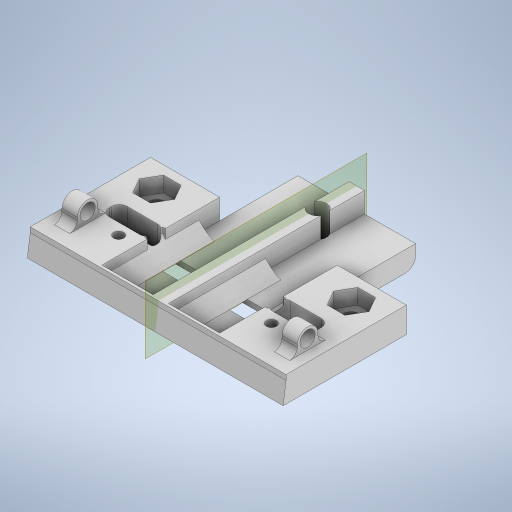
# Autodesk Inventor part: podsta
Saved by Autodesk Inventor 2023 (Build 270158000, 158)
## iProperties
Created: 2022-12-13
Part Number: podsta
Material: Generic
Document SubType Name: Modeling
Designer: komputer
Density: 1 g/cm^3
Appearance: Default
Author: komputer
Autodesk Inventor part; units mm, degrees
ref_plane "YZ Plane" through (0, 0, 0) normal (1, 0, 0) x (0, 1, 0)
ref_plane "XZ Plane" through (0, 0, 0) normal (0, 1, 0) x (-1, 0, 0)
ref_plane "XY Plane" through (0, 0, 0) normal (0, 0, 1) x (1, 0, 0)
sketch "Sketch1" plane through (0, 0, 0) normal (0, 1, 0) x (-1, 0, 0)
  line L0 (-25, -25) -> (25, -25)
  line L1 (25, -25) -> (25, 25)
  line L2 (25, 25) -> (-25, 25)
  line L3 (-25, 25) -> (-25, -25)
  point P0 (0, 0)
  dimension "d2" = 50
  dimension "d3" = 50
  constraints: 8 end point, 2 parallel, 1 horizontal, 1 perpendicular
  measures "d2" distance of L2.end L1.end
  measures "d3" distance of L1.end L0.end
extrude "Extrusion1" add sketch "Sketch1" along normal blind 4
sketch "Sketch2" plane through (0, 4, 0) normal (0, 1, 0) x (1, 0, 0)
  line L0 (-25, 25) -> (-25, -25) projected
  line L1 (-25, -25) -> (25, -25) projected
  line L2 (25, -25) -> (25, 25) projected
  line L3 (25, 25) -> (-25, 25) projected
  line L4 (-25, -25) -> (25, -25) projected
  line L5 (0, -25) -> (0, 25)
  line L6 (25, 25) -> (-25, 25) projected
  line L7 (0, -25) -> (-1.5, -25)
  line L8 (-1.5, -25) -> (1.5, -25)
  line L9 (1.5, -25) -> (1.5, 25)
  line L10 (1.5, 25) -> (-1.5, 25)
  line L11 (-1.5, 25) -> (-1.5, -25)
  line L12 (1.5, 9.2284) -> (-1.5, 9.2284)
  line L13 (1.5, 9.2284) -> (-1.5, 9.2284)
  line L14 (-1.5, 9.2284) -> (-1.5, 25)
  line L15 (-1.5, 25) -> (1.5, 25)
  line L16 (1.5, 25) -> (1.5, 9.2284)
  point P0 (0, 0)
  point P1 (1.5, 25)
  dimension "d6" = 1.5
  dimension "d7" = 3
  constraints: 22 end point, 4 parallel, 4 point on line, 3 perpendicular, 2 horizontal, 2 midpoint
  measures "d6" distance of L5.start L7.end
  measures "d7" distance of L10.end L9.end
extrude "Extrusion2" add sketch "Sketch2" along normal blind 3 contours L3 L5 L12 L11 | L3 L9 L12 L5
sketch "Sketch3" plane through (0, 4, 0) normal (0, 1, 0) x (1, 0, 0)
  line L0 (1.5, 25) -> (1.5, 9.2284) projected
  line L1 (1.5, 9.2284) -> (-1.5, 9.2284) projected
  line L2 (-1.5, 9.2284) -> (-1.5, 25) projected
  line L3 (-1.5, 25) -> (-25, 25) projected
  line L4 (-25, 25) -> (-25, -25) projected
  line L5 (-25, -25) -> (25, -25) projected
  line L6 (25, -25) -> (25, 25) projected
  line L7 (25, 25) -> (1.5, 25) projected
  line L8 (11.5, 24.5) -> (11.5, 9.7) projected
  line L9 (-11.5, 9.7) -> (-11.5, 24.5) projected
  line L10 (25, 25) -> (1.5, 25) projected
  line L11 (25, 25) -> (11.5, 25)
  line L12 (11.5, 25) -> (11.5, 9.7)
  line L13 (11.5, 9.7) -> (25, 9.7)
  line L14 (25, 9.7) -> (25, 25)
  line L15 (-11.5, 9.7) -> (-25, 9.7)
  line L16 (-25, 9.7) -> (-25, 25)
  line L17 (-25, 25) -> (-11.5, 25)
  line L18 (-11.5, 25) -> (-11.5, 9.7)
  point P0 (0, 0)
  constraints: 16 end point, 4 parallel, 2 horizontal, 2 perpendicular
extrude "Extrusion3" cut sketch "Sketch3" against normal blind 10 contours L7 L6 L13 L8 L12 | L18 L9 L15 L4 L3
sketch "Sketch4" plane through (0, 0, 0) normal (0, -1, 0) x (1, 0, 0)
  line L0 (-11.5, -9.7) -> (-11.5, -25) projected
  line L1 (11.5, -25) -> (-11.5, -25) projected
  line L2 (11.5, -25) -> (11.5, -9.7) projected
  line L3 (11.5, -9.7) -> (25, -9.7) projected
  line L4 (25, 25) -> (25, -9.7) projected
  line L5 (-25, 25) -> (25, 25) projected
  line L6 (-25, -9.7) -> (-25, 25) projected
  line L7 (-25, -9.7) -> (-11.5, -9.7) projected
  point P0 (0, 0)
extrude "Extrusion4" cut sketch "Sketch4" against normal blind 1
sketch "Sketch5" plane through (-25, 4, 25) normal (0, 0, 1) x (1, 0, 0)
  line L0 (0, -3) -> (50, -3) projected
  line L1 (50, -3) -> (50, 0) projected
  line L2 (0, 0) -> (50, 0) projected
  line L3 (0, -3) -> (0, 0) projected
  line L4 (0, 0) -> (50, 0) projected
  line L5 (0, 0) -> (50, 0)
  line L6 (50, 0) -> (50, 3)
  line L7 (50, 3) -> (0, 3)
  line L8 (0, 3) -> (0, 0)
  point P0 (25, -4)
  dimension "d14" = 3
  constraints: 8 end point, 2 parallel, 1 horizontal, 1 perpendicular
  measures "d14" distance of L6.end L5.end
extrude "Extrusion5" add sketch "Sketch5" against normal up to surface (34.7 mm away) contours L8 L7 L6 L2
sketch "Sketch6" plane through (11.5, 4, -9.7) normal (0, 0, -1) x (-1, 0, 0)
  line L0 (-13.5, -3) -> (0, -3) projected
  line L1 (0, 0) -> (0, -3) projected
  line L2 (10, 0) -> (0, 0) projected
  line L3 (10, 3) -> (10, 0) projected
  line L4 (10, 3) -> (-13.5, 3) projected
  line L5 (-13.5, -3) -> (-13.5, 3) projected
  line L6 (23, -3) -> (36.5, -3) projected
  line L7 (36.5, 3) -> (36.5, -3) projected
  line L8 (36.5, 3) -> (13, 3) projected
  line L9 (13, 0) -> (13, 3) projected
  line L10 (23, 0) -> (13, 0) projected
  line L11 (23, 0) -> (23, -3) projected
  line L12 (0, 0.5) -> (0, 11.5) projected
  line L13 (23, 11.5) -> (23, 0.5) projected
  line L14 (10, 0) -> (0, 0) projected
  line L15 (0, 11.5) -> (0, 0)
  line L16 (23, 11.5) -> (23, 0)
  line L17 (0, 0) -> (0, -3) projected
  line L18 (10, 3) -> (-13.5, 3) projected
  line L19 (0, 0) -> (10, 0)
  line L20 (10, 0) -> (10, 3)
  line L21 (10, 3) -> (0, 3)
  line L22 (0, 3) -> (0, 0)
  line L23 (13, 0) -> (13, 3) projected
  line L24 (23, 0) -> (23, -3) projected
  line L25 (13, 3) -> (23, 3)
  line L26 (23, 3) -> (23, 0)
  line L27 (23, 0) -> (13, 0)
  line L28 (13, 0) -> (13, 3)
  point P0 (11.5, -4)
  point P1 (23, 0.5)
  point P2 (0, 3)
  constraints: 20 end point, 4 parallel, 3 perpendicular, 2 horizontal, 1 vertical
extrude "Extrusion6" cut sketch "Sketch6" against normal blind 20 contours L15 L12 L4 L3 L2 | L10 L9 L8 L13 L16
sketch "Sketch7" plane through (11.5, 4, 10.3) normal (0, 0, -1) x (-1, 0, 0)
  arc A0 (0, 2.75) -> (10, 2.7503) centre (4.9999, 5.9206) ccw projected
  arc A1 (13, 2.75) -> (23, 2.7497) centre (18.0001, 5.9203) ccw projected
  line L0 (0, 0) -> (10, 0) projected
  line L1 (5, 0) -> (5, -0.3289)
  line L2 (5, -0.3289) -> (19.1354, -0.3289)
  circle A2 centre (4.9999, 5.9206) radius 6.2495
  circle A3 centre (18.0001, 5.9203) radius 6.2492
  line L3 (0, 3) -> (-13.5, 3) projected
  line L4 (0, 3) -> (10, 3)
  line L5 (10, 3) -> (10, 0)
  line L6 (10, 0) -> (0, 0)
  line L7 (0, 0) -> (0, 3)
  line L8 (13, 0) -> (13, 3) projected
  line L9 (23, 3) -> (23, 0) projected
  line L10 (13, 0) -> (23, 0)
  line L11 (23, 0) -> (23, 3)
  line L12 (23, 3) -> (13, 3)
  line L13 (13, 3) -> (13, 0)
  point P0 (11.5, -4)
  point P1 (20.0008, 0)
  point P2 (23, 2.1715)
  point P3 (15.9994, 0)
  point P4 (13, 2.1717)
  point P5 (10, 2.1715)
  point P6 (7.0007, 0)
  point P7 (0, 2.1713)
  point P8 (2.9992, 0)
  constraints: 20 end point, 4 parallel, 3 perpendicular, 2 coincident, 2 horizontal, 1 centre point, 1 midpoint, 1 tangent, 1 vertical, 3 other
extrude "Extrusion7" add sketch "Sketch7" along normal blind 16 contours A2 L0 L7 | A2 L5 L0 | A3 L10 L8 | A3 L9 L10
chamfer "Chamfer1" distance 3 angle 45 2 edges at (6.5, 7, 10.3) (-6.5, 7, 10.3)
sketch "Sketch8" plane through (-25, 7, -9.7) normal (-1, 0, 0) x (0, 0, 1)
  circle A0 centre (-11.34, 3) radius 8 projected
  line L0 (0, -6) -> (34.7, -6) projected
  line L1 (34.7, -6) -> (34.7, 0) projected
  line L2 (34.7, 0) -> (0, 0) projected
  line L3 (0, 0) -> (0, -6) projected
  line L4 (-11.34, 3) -> (-19.34, 3)
  line L5 (-19.34, 3) -> (-22.34, 3)
  line L6 (-22.34, 3) -> (27.66, 3)
  line L7 (0, -6) -> (34.7, -6) projected
  line L8 (34.7, -6) -> (27.66, -6)
  line L9 (27.66, -6) -> (27.66, 9.5427)
  line L10 (27.66, 9.5427) -> (34.7, 9.5427)
  line L11 (34.7, 9.5427) -> (34.7, -6)
  point P0 (9.7, -7)
  point P1 (27.66, 0)
  dimension "d24" = 3
  dimension "d25" = 50
  constraints: 14 end point, 2 parallel, 2 point on line, 1 horizontal, 1 horizontal alignment, 1 perpendicular, 1 other
  measures "d24" distance of L4.end L5.end
  measures "d25" distance of L5.end L6.end
extrude "Extrusion8" cut sketch "Sketch8" against normal through all contours L9 L2 L1 L0
sketch "Sketch9" plane through (25, 1, -9.7) normal (1, 0, 0) x (0, 0, -1)
  line L0 (-27.66, 6) -> (-27.66, 0) projected
  line L1 (-27.66, 0) -> (0, 0) projected
  line L2 (0, 0) -> (0, 6) projected
  line L3 (-27.66, 6) -> (0, 6) projected
  line L4 (-27.66, 0.31) -> (-25.7682, 0.01) projected
  line L5 (-25.7682, 0.01) -> (-14.0234, 0.01) projected
  line L6 (-14.0234, 0.01) -> (-14.0234, 0.61) projected
  line L7 (-25.7682, 0.61) -> (-14.0234, 0.61) projected
  line L8 (-25.7682, 0.61) -> (-27.66, 0.31) projected
  line L9 (-27.66, 0) -> (-27.66, 6) projected
  line L10 (-14.0234, 0.61) -> (-27.66, 0.61)
  line L11 (-27.66, 0.61) -> (-27.66, 1.22)
  line L12 (-27.66, 1.22) -> (-14.0234, 1.22)
  line L13 (-14.0234, 1.22) -> (-14.0234, 0.61)
  point P0 (-9.7, -1)
  point P1 (-27.66, 1.22)
  dimension "d28" = 0.61
  constraints: 8 end point, 2 parallel, 1 horizontal, 1 perpendicular, 1 point on line, 1 other
  measures "d28" distance of L10.end L11.end
extrude "Extrusion9" cut sketch "Sketch9" against normal through all contours L12 L13 L7 L10 L0
sketch "Sketch10" plane through (25, 1, -9.7) normal (1, 0, 0) x (0, 0, -1)
  line L0 (-27.66, 0.31) -> (-25.7682, 0.01) projected
  line L1 (-25.7682, 0.01) -> (-14.0234, 0.01) projected
  line L2 (-14.0234, 0.01) -> (-14.0234, 0.61) projected
  line L3 (-25.7682, 0.61) -> (-14.0234, 0.61) projected
  line L4 (-25.7682, 0.61) -> (-27.66, 0.31) projected
  line L5 (-14.0234, 1.22) -> (-14.0234, 0.61) projected
  line L6 (-27.66, 0) -> (0, 0) projected
  line L7 (0, 0) -> (0, 6) projected
  line L8 (-27.66, 6) -> (0, 6) projected
  line L9 (-27.66, 6) -> (-27.66, 1.22) projected
  line L10 (-27.66, 1.22) -> (-14.0234, 1.22) projected
  line L11 (-25.7682, 0.61) -> (-25.7682, 6)
  line L12 (-27.66, 6) -> (0, 6) projected
  line L13 (-19.9, 5.7) -> (-19.9, 6.1)
  line L14 (15.3, 6) -> (-23, 6) projected
  line L15 (-19.9, 6) -> (-20.9, 6)
  line L16 (-20.9, 6) -> (-23.9, 6)
  line L17 (-25.7682, 0.61) -> (-23.9, 6)
  line L18 (-14.0234, 0.61) -> (-27.66, 0.61) projected
  line L19 (-27.66, 0.61) -> (-27.66, 0) projected
  point P0 (-9.7, -1)
  point P1 (-25.5568, 1.22)
  dimension "d31" = 1
  dimension "d32" = 3
  constraints: 10 end point, 5 point on line, 1 perpendicular, 1 vertical, 2 other
  measures "d31" distance of L15.start L15.end
  measures "d32" distance of L15.end L16.end
extrude "Extrusion10" cut sketch "Sketch10" against normal through all contours L11 L8 L17 L10 | L10 L9 L8 L11
sketch "Sketch11" plane through (0, 1, 0) normal (0, -1, 0) x (1, 0, 0)
  circle A0 centre (0, -17.35) radius 1.5 projected
  line L0 (3.695, -17.35) -> (1.8475, -14.15) projected
  line L1 (1.8475, -20.55) -> (3.695, -17.35) projected
  line L2 (-1.8475, -20.55) -> (1.8475, -20.55) projected
  line L3 (-3.695, -17.35) -> (-1.8475, -20.55) projected
  line L4 (-1.8475, -14.15) -> (-3.695, -17.35) projected
  line L5 (1.8475, -14.15) -> (-1.8475, -14.15) projected
  circle A1 centre (0, -17.35) radius 1.5 projected
  line L6 (-25, -10.04) -> (-25, -32.04) projected
  point P0 (0, 0)
extrude "Extrusion11" cut sketch "Sketch11" against normal through all contours A0
chamfer "Chamfer2" distance 1 angle 45 1 edges at (-1.5, 1, -17.35)
sketch "Sketch12" plane through (-25, 1, -9.7) normal (-1, 0, 0) x (0, 0, 1)
  line L0 (25.5568, 1.22) -> (23.9, 6) projected
  line L1 (23.9, 6) -> (0, 6) projected
  line L2 (0, 6) -> (0, 0) projected
  line L3 (0, 0) -> (27.66, 0) projected
  line L4 (27.66, 0) -> (27.66, 0.61) projected
  line L5 (27.66, 0.61) -> (14.0234, 0.61) projected
  line L6 (14.0234, 0.61) -> (14.0234, 1.22) projected
  line L7 (14.0234, 1.22) -> (25.5568, 1.22) projected
  circle A0 centre (-11.34, 9) radius 11 projected
  line L8 (-22.34, 9) -> (27.66, 9)
  line L9 (27.66, 9) -> (27.66, -12.93)
  line L10 (-11.34, 9) -> (-11.34, -2)
  line L11 (-11.34, -2) -> (27.66, -1.965)
  line L12 (14.0234, 1.22) -> (25.5568, 1.22) projected
  line L13 (27.66, -1.3745) -> (14.0234, 1.22)
  line L14 (14.0234, 1.22) -> (14.0795, 1.5147)
  line L15 (14.0234, 1.22) -> (13.9673, 0.9253)
  line L16 (14.0795, 1.5147) -> (28.9229, -1.3094)
  line L17 (13.9673, 0.9253) -> (29.035, -1.9638)
  line L18 (25.5568, 1.22) -> (24.566, 4.0785)
  line L19 (25.5568, 1.22) -> (23.9, 6) projected
  line L20 (25.5568, 1.22) -> (26.2577, -0.8023)
  point P0 (9.7, -1)
  point P1 (15.6117, 0.61)
  point P2 (14.0234, 0.9145)
  point P3 (15.6285, 1.22)
  dimension "d40" = 0.3
  dimension "d41" = 0.3
  constraints: 22 end point, 4 point on line, 2 perpendicular, 2 point on circle, 2 vertical, 1 horizontal, 1 midpoint, 1 parallel
  measures "d40" distance of L6.end L14.end
  measures "d41" distance of L6.end L15.end
extrude "Extrusion12" add sketch "Sketch12" against normal blind 50 contours L20 L5 L16 L7 | L20 L3 L16 L5 | L20 L16 L3 | L17 L5 L6
sketch "Sketch13" plane through (-25, 1, -9.7) normal (-1, 0, 0) x (0, 0, 1)
  line L0 (18.8347, 0.61) -> (15.6117, 0.61) projected
  line L1 (15.6117, 0.61) -> (14.0234, 0.9145) projected
  line L2 (14.0234, 0.9145) -> (14.0234, 1.22) projected
  line L3 (14.0234, 1.22) -> (15.6285, 1.22) projected
  line L4 (15.6285, 1.22) -> (18.8347, 0.61) projected
  line L5 (25.7682, 0.61) -> (23.9, 6) projected
  line L6 (23.9, 6) -> (0, 6) projected
  line L7 (0, 6) -> (0, 0) projected
  line L8 (0, 0) -> (22.0408, 0) projected
  line L9 (22.0408, 0) -> (26.2577, -0.8023) projected
  line L10 (26.2577, -0.8023) -> (25.9796, 0) projected
  line L11 (25.9796, 0) -> (27.66, 0) projected
  line L12 (27.66, 0) -> (27.66, 0.61) projected
  line L13 (27.66, 0.61) -> (25.7682, 0.61) projected
  line L14 (14.0234, 0.9145) -> (14.0234, 1.22) projected
  line L15 (14.0234, 0.9145) -> (26.7141, -1.5188)
  line L16 (14.0234, 1.22) -> (15.6285, 1.22) projected
  line L17 (15.6285, 1.22) -> (29.31, -1.383)
  line L18 (14.0234, 0.9145) -> (13.2268, 1.0673)
  line L19 (13.2268, 1.0673) -> (13.3704, 1.8159)
  line L20 (15.6285, 1.22) -> (13.3396, 1.6555)
  line L21 (25.9796, 0) -> (27.66, 0) projected
  line L22 (25.9796, 0) -> (25.7682, 0.61)
  line L23 (26.7141, -1.5188) -> (27.0047, -0.9444)
  point P0 (9.7, -1)
  point P1 (18.7931, 0)
  constraints: 14 end point, 3 point on line, 1 perpendicular
extrude "Extrusion13" cut sketch "Sketch13" against normal through all contours L17 L8 L15 L0 | L3 L2 L18 L19 L20 | L22 L13 L12 L11
sketch "Sketch14" plane through (-25, 1, -9.7) normal (-1, 0, 0) x (0, 0, 1)
  line L0 (26.2577, -0.8023) -> (23.9, 6) projected
  line L1 (23.9, 6) -> (0, 6) projected
  line L2 (0, 6) -> (0, 0) projected
  line L3 (0, 0) -> (18.7931, 0) projected
  line L4 (18.7931, 0) -> (13.2268, 1.0673) projected
  line L5 (13.2268, 1.0673) -> (13.3396, 1.6555) projected
  line L6 (13.3396, 1.6555) -> (26.2577, -0.8023) projected
  circle A0 centre (-11.34, 9) radius 11 projected
  line L7 (-22.34, 9) -> (27.66, 9)
  line L8 (-11.34, 9) -> (-11.34, -2)
  line L9 (-11.34, 9) -> (27.66, 9)
  line L10 (27.66, 9) -> (27.66, -2)
  line L11 (27.66, -2) -> (-11.34, -2)
  line L12 (-11.34, -2) -> (-11.34, 9)
  line L13 (4, 3) -> (-7.65, 3) projected
  line L14 (-7.65, 3) -> (-15.3, 3) projected
  line L15 (-15.3, 3) -> (0, 3) projected
  line L16 (0, 3) -> (4, 3) projected
  line L17 (4, 3) -> (20, 3) projected
  line L18 (20, 3) -> (4, 3) projected
  line L19 (0, 3) -> (-15.3, 3) projected
  line L20 (0, 3) -> (20, 3)
  line L21 (20, 3) -> (20, 2)
  line L22 (20, 2) -> (0, 2)
  line L23 (0, 2) -> (0, 3)
  line L24 (22.1715, 5.1715) -> (20, 3) projected
  line L25 (20, 3) -> (29.0462, 3)
  line L26 (29.0462, 3) -> (29.0462, 2)
  line L27 (29.0462, 2) -> (20, 2)
  line L28 (20, 2) -> (20, 3)
  line L29 (27.66, 2) -> (-2.34, 2)
  line L30 (-2.34, 2) -> (-2.34, -1)
  line L31 (-2.34, -1) -> (27.66, -1)
  line L32 (27.66, -1) -> (27.66, 2)
  line L33 (27.66, -1) -> (24.0847, 2)
  line L34 (26.2577, -0.8023) -> (23.9, 6) projected
  line L35 (24.0847, 2) -> (23.5108, 6)
  line L36 (23.9, 6) -> (0, 6) projected
  point P0 (9.7, -1)
  point P1 (24.0847, 2)
  point P2 (25.7792, 0.5781)
  dimension "d46" = 50
  dimension "d47" = 1
  dimension "d48" = 30
  dimension "d49" = 3
  dimension "d50" = 40
  constraints: 40 end point, 8 parallel, 5 horizontal, 5 point on line, 4 perpendicular, 2 point on circle, 1 vertical
  measures "d46" distance of L7.start L7.end
  measures "d47" distance of L20.end L21.end
  measures "d48" distance of L31.end L30.end
  measures "d49" distance of L30.end L29.end
  measures "d50" angle of L31 L33
extrude "Extrusion14" cut sketch "Sketch14" against normal through all contours L6 L5 L4 L3 L2 L22 L27 L33 L0 | L0 L33 L31 L30 L29 L2 L3 L4 L5 L6 | L33 L27 L0 | L27 L35 L25 L0 | L25 L35 L1 L0
sketch "Szkic15" plane through (-25, 3, -9.7) normal (0, -1, 0) x (1, 0, 0)
  line L0 (4.5, 10.603) -> (4.5, 23.16) projected
  line L1 (4.5, 23.16) -> (15.406, 23.16) projected
  line L2 (15.406, 23.16) -> (15.406, 10.603) projected
  line L3 (15.406, 10.603) -> (4.5, 10.603) projected
  line L4 (34.594, 10.603) -> (34.594, 23.16) projected
  line L5 (34.594, 23.16) -> (45.5, 23.16) projected
  line L6 (45.5, 23.16) -> (45.5, 10.603) projected
  line L7 (45.5, 10.603) -> (34.594, 10.603) projected
  line L8 (0, -2.34) -> (0, 27.66) projected
  line L9 (0, -2.34) -> (50, -2.34) projected
  line L10 (50, 27.66) -> (50, -2.34) projected
  line L11 (0, 27.66) -> (50, 27.66) projected
  circle A0 centre (39.92, 16.31) radius 1 projected
  line L12 (25, 27.66) -> (25, -2.34)
  line L13 (36.5, -2.34) -> (13.5, -2.34) projected
  circle A1 centre (10.08, 16.31) radius 1
  circle A2 centre (44, 3) radius 1.75
  circle A3 centre (6, 3) radius 1.75
  circle A4 centre (6, 4.75) radius 1.5 projected
  circle A5 centre (44, 4.75) radius 1.5 projected
  point P0 (25, 9.7)
  dimension "d53" = 3.5
  dimension "d54" = 3.5
  constraints: 3 centre point, 2 end point, 2 midpoint, 1 symmetric about line, 1 other
  measures "d53" diameter of A2
  measures "d54" diameter of A3
extrude "Wyciągnięcie proste15" cut sketch "Szkic15" against normal through all contours A0 | A1 | A2 A5 | A5 A2 | A3 A4 | A4 A3 picked at (44.0188, 1.9252) picked at (44.24, 4.2484) picked at (6.0188, 1.9252) picked at (5.76, 4.2484)
sketch "Szkic16" plane through (-25, 3, -9.7) normal (0, -1, 0) x (1, 0, 0)
  circle A0 centre (6, 3) radius 1.75 projected
  circle A1 centre (44, 3) radius 1.75 projected
  point P0 (25, 9.7)
extrude "Wyciągnięcie proste16" add sketch "Szkic16" against normal up to surface (4 mm away)
sketch "Szkic17" plane through (-25, 3, -9.7) normal (0, -1, 0) x (1, 0, 0)
  circle A0 centre (44, 4.75) radius 1.5 projected
  circle A1 centre (6, 4.75) radius 1.5 projected
  circle A2 centre (44, 4.75) radius 1.75
  circle A3 centre (6, 4.75) radius 1.75
  point P0 (25, 9.7)
  dimension "d59" = 3.5
  dimension "d60" = 3.5
  constraints: 2 centre point, 2 coincident
  measures "d59" diameter of A2
  measures "d60" diameter of A3
extrude "Wyciągnięcie proste17" cut sketch "Szkic17" against normal through all contours A0 | A1 | A2 | A3
sketch "Szkic19" plane through (-25, 3, -9.7) normal (0, -1, 0) x (1, 0, 0)
  line L0 (15.406, 10.603) -> (4.5, 10.603) projected
  line L1 (15.406, 23.16) -> (15.406, 10.603) projected
  line L2 (4.5, 10.603) -> (4.5, 23.16) projected
  line L3 (45.5, 10.603) -> (34.594, 10.603) projected
  line L4 (45.5, 23.16) -> (45.5, 10.603) projected
  line L5 (34.594, 10.603) -> (34.594, 23.16) projected
  line L6 (4.5, 23.16) -> (15.406, 23.16) projected
  line L7 (34.594, 23.16) -> (45.5, 23.16) projected
  line L8 (15.406, 10.603) -> (4.5, 10.603)
  line L9 (4.5, 10.603) -> (4.5, 14.1211)
  line L10 (4.5, 14.1211) -> (15.406, 14.1211)
  line L11 (15.406, 14.1211) -> (15.406, 10.603)
  line L12 (15.406, 14.1211) -> (45.5, 14.1211)
  line L13 (45.5, 14.1211) -> (45.5, 10.603)
  line L14 (45.5, 10.603) -> (15.406, 10.603)
  line L15 (15.406, 10.603) -> (15.406, 14.1211)
  line L16 (13.5, 23) -> (13.5, 0) projected
  line L17 (36.5, 0) -> (36.5, 23) projected
  point P0 (25, 9.7)
  point P1 (13.5, 10.603)
  point P2 (13.5, 14.1211)
  point P3 (36.5, 14.1211)
  point P4 (36.5, 10.603)
  constraints: 16 end point, 4 parallel, 2 horizontal, 2 perpendicular, 1 point on line
extrude "Wyciągnięcie proste18" cut sketch "Szkic19" against normal through all contours L0 L2 L10 L16 | L17 L12 L4 L3
fillet "Zaokrąglenie1" radius 1.5 8 edges at (20.5, 5, 0.903) (20.5, 5, 4.4211) (-20.5, 5, 4.4211) (-20.5, 5, 0.903) (11.5, 4.5856, 0.903) (11.5, 4.5856, 4.4211) (-11.5, 4.5857, 0.903) (-11.5, 4.5857, 4.4211)
sketch "Szkic20" plane through (-25, 3, -9.7) normal (0, -1, 0) x (1, 0, 0)
  line L0 (4.5, 12.103) -> (4.5, 12.6211) projected
  arc A0 (6, 14.1211) -> (4.5, 12.6211) centre (6, 12.6211) ccw projected
  line L1 (6, 14.1211) -> (12, 14.1211) projected
  arc A1 (13.5, 12.6211) -> (12, 14.1211) centre (12, 12.6211) ccw projected
  line L2 (13.5, 12.6211) -> (13.5, 12.103) projected
  arc A2 (12, 10.603) -> (13.5, 12.103) centre (12, 12.103) ccw projected
  line L3 (12, 10.603) -> (6, 10.603) projected
  arc A3 (4.5, 12.103) -> (6, 10.603) centre (6, 12.103) ccw projected
  line L4 (45.5, 12.6211) -> (45.5, 12.103) projected
  arc A4 (44, 10.603) -> (45.5, 12.103) centre (44, 12.103) ccw projected
  line L5 (44, 10.603) -> (38, 10.603) projected
  arc A5 (36.5, 12.103) -> (38, 10.603) centre (38, 12.103) ccw projected
  line L6 (36.5, 12.103) -> (36.5, 12.6211) projected
  arc A6 (38, 14.1211) -> (36.5, 12.6211) centre (38, 12.6211) ccw projected
  line L7 (38, 14.1211) -> (44, 14.1211) projected
  arc A7 (45.5, 12.6211) -> (44, 14.1211) centre (44, 12.6211) ccw projected
  circle A8 centre (6, 4.75) radius 1.75 projected
  circle A9 centre (44, 4.75) radius 1.75 projected
  circle A10 centre (10.08, 16.31) radius 1 projected
  circle A11 centre (39.92, 16.31) radius 1 projected
  line L8 (36.5, 0) -> (36.5, -2.34) projected
  line L9 (50, 0) -> (36.5, 0) projected
  line L10 (50, 24.0847) -> (50, 0) projected
  line L11 (0, 24.0847) -> (50, 24.0847) projected
  line L12 (0, 0) -> (0, 24.0847) projected
  line L13 (13.5, 0) -> (0, 0) projected
  line L14 (13.5, -2.34) -> (13.5, 0) projected
  line L15 (13.5, -2.34) -> (36.5, -2.34) projected
  line L16 (44, 14.1211) -> (38, 14.1211) projected
  line L17 (12, 14.1211) -> (38, 14.1211)
  line L18 (12, 10.603) -> (38, 10.603)
  point P0 (25, 9.7)
  constraints: 4 end point, 1 collinear, 1 horizontal
extrude "Wyciągnięcie proste19" cut sketch "Szkic20" against normal blind 1 contours A2 L2 A1 L17 A6 L6 A5 L18
sketch "Szkic21" plane through (0, 1, 0) normal (0, -1, 0) x (1, 0, 0)
  line L0 (11.5, -12.04) -> (-11.5, -12.04) projected
  line L1 (-11.5, -25) -> (-11.5, -12.04) projected
  line L2 (11.5, -25) -> (-11.5, -25) projected
  line L3 (11.5, -12.04) -> (11.5, -25) projected
  circle A0 centre (0, -17.35) radius 2.5 projected
  point P0 (0, 0)
ref_plane "Płaszczyzna konstrukcyjna1" through (-25, 0, -12.04) normal (0, -1, 0) x (1, 0, 0)
extrude "Wyciągnięcie proste20" add sketch "Szkic21" along normal up to surface (1 mm away)
fillet "Zaokrąglenie2" radius 2 1 edges at (0, 0, -25)
sketch "Szkic22" plane through (0, 7, 0) normal (0, 1, 0) x (1, 0, 0)
  arc A0 (-1.5, 17.35) -> (1.5, 17.35) centre (0, 17.35) ccw projected
  circle A1 centre (0, 17.35) radius 1.75
  point P0 (0, 0)
  dimension "d71" = 3.5
  constraints: 1 centre point, 1 coincident
  measures "d71" diameter of A1
extrude "Wyciągnięcie proste21" cut sketch "Szkic22" against normal through all
sketch "Szkic23" plane through (-11.5, 0, -12.04) normal (0, -1, 0) x (1, 0, 0)
  circle A0 centre (11.5, -5.31) radius 1.75 projected
  line L0 (23, -10.96) -> (0, -10.96) projected
  line L1 (23, 0) -> (23, -10.96) projected
  line L2 (0, 0) -> (23, 0) projected
  line L3 (0, -10.96) -> (0, 0) projected
  circle A1 centre (11.5, -5.31) radius 2.5 projected
  point P0 (11.5, 12.04)
extrude "Wyciągnięcie proste22" add sketch "Szkic23" against normal blind 2 contours A1
chamfer "Faza3" distance 1.5 angle 45 1 edges at (-1.75, 0, -17.35)
sketch "Szkic24" plane through (0, 7, 0) normal (0, 1, 0) x (1, 0, 0)
  circle A0 centre (14.92, -6.61) radius 1 projected
  circle A1 centre (-14.92, -6.61) radius 1 projected
  circle A2 centre (19, 4.95) radius 1.75 projected
  circle A3 centre (-19, 4.95) radius 1.75 projected
  arc A4 (-1.5, 16.4486) -> (1.5, 16.4486) centre (0, 17.35) ccw projected
  line L0 (-1.5, 16.4486) -> (-1.5, -13.3) projected
  line L1 (-11.5, -13.3) -> (-1.5, -13.3) projected
  line L2 (-11.5, -13.3) -> (-11.5, -4.4211) projected
  line L3 (-11.5, -4.4211) -> (-12.025, -4.4211) projected
  line L4 (-12.025, -4.061) -> (-12.025, -4.4211) projected
  arc A5 (-13, -4.4211) -> (-12.025, -4.061) centre (-13, -2.9211) ccw projected
  line L5 (-13, -4.4211) -> (-19, -4.4211) projected
  arc A6 (-20.5, -2.9211) -> (-19, -4.4211) centre (-19, -2.9211) ccw projected
  line L6 (-20.5, -2.9211) -> (-20.5, -2.403) projected
  arc A7 (-19, -0.903) -> (-20.5, -2.403) centre (-19, -2.403) ccw projected
  line L7 (-19, -0.903) -> (-13, -0.903) projected
  arc A8 (-12.025, -1.2631) -> (-13, -0.903) centre (-13, -2.403) ccw projected
  line L8 (-12.025, -1.2631) -> (-12.025, -0.903) projected
  line L9 (-12.025, -0.903) -> (-11.5, -0.903) projected
  line L10 (-11.5, -0.903) -> (-11.5, 9.7) projected
  line L11 (-25, 9.7) -> (-11.5, 9.7) projected
  line L12 (-25, -13.8108) -> (-25, 9.7) projected
  line L13 (-25, -13.8108) -> (25, -13.8108) projected
  line L14 (25, -13.8108) -> (25, 9.7) projected
  line L15 (11.5, 9.7) -> (25, 9.7) projected
  line L16 (11.5, 9.7) -> (11.5, -0.903) projected
  line L17 (11.5, -0.903) -> (12.0252, -0.903) projected
  line L18 (12.0252, -1.263) -> (12.0252, -0.903) projected
  arc A9 (13, -0.903) -> (12.0252, -1.263) centre (13, -2.403) ccw projected
  line L19 (13, -0.903) -> (19, -0.903) projected
  arc A10 (20.5, -2.403) -> (19, -0.903) centre (19, -2.403) ccw projected
  line L20 (20.5, -2.403) -> (20.5, -2.9211) projected
  arc A11 (19, -4.4211) -> (20.5, -2.9211) centre (19, -2.9211) ccw projected
  line L21 (19, -4.4211) -> (13, -4.4211) projected
  arc A12 (12.0252, -4.0612) -> (13, -4.4211) centre (13, -2.9211) ccw projected
  line L22 (12.0252, -4.0612) -> (12.0252, -4.4211) projected
  line L23 (12.0252, -4.4211) -> (11.5, -4.4211) projected
  line L24 (11.5, -4.4211) -> (11.5, -13.3) projected
  line L25 (1.5, -13.3) -> (11.5, -13.3) projected
  line L26 (1.5, -13.3) -> (1.5, 16.4486) projected
  line L27 (19, 4.95) -> (19, 7.95)
  line L28 (0, -13.8108) -> (0, -18.7372)
  circle A13 centre (19, 4.95) radius 1.75 projected
  line L29 (20.7321, 7.95) -> (22.4641, 4.95)
  line L30 (22.4641, 4.95) -> (20.7321, 1.95)
  line L31 (20.7321, 1.95) -> (17.2679, 1.95)
  line L32 (17.2679, 1.95) -> (15.5359, 4.95)
  line L33 (15.5359, 4.95) -> (17.2679, 7.95)
  line L34 (17.2679, 7.95) -> (20.7321, 7.95)
  circle A14 centre (-19, 4.95) radius 1.75 projected
  line L35 (-17.2679, 7.95) -> (-15.5359, 4.95)
  line L36 (-15.5359, 4.95) -> (-17.2679, 1.95)
  line L37 (-17.2679, 1.95) -> (-20.7321, 1.95)
  line L38 (-20.7321, 1.95) -> (-22.4641, 4.95)
  line L39 (-22.4641, 4.95) -> (-20.7321, 7.95)
  line L40 (-20.7321, 7.95) -> (-17.2679, 7.95)
  point P0 (0, 0)
  point P1 (-19, 7.95)
  dimension "d79" = 3
  constraints: 28 end point, 3 midpoint, 2 coincident, 2 vertical, 1 point on line, 26 other
  measures "d79" distance of L27.start L27.end
extrude "Wyciągnięcie proste23" add sketch "Szkic24" along normal blind 1 contours A4 L26 L25 L24 L23 L22 A12 L21 A11 L20 A10 L19 A9 L18 L17 L16 L15 L14 L13 L12 L11 L10 L9 L8 A8 L7 A7 L6 A6 L5 A5 L4 L3 L2 L1 L0
sketch "Szkic25" plane through (0, 7, 0) normal (0, 1, 0) x (1, 0, 0)
  circle A0 centre (-19, 4.95) radius 1.75 projected
  line L0 (-17.2679, 7.95) -> (-20.7321, 7.95) projected
  line L1 (-20.7321, 7.95) -> (-22.4641, 4.95) projected
  line L2 (-22.4641, 4.95) -> (-20.7321, 1.95) projected
  line L3 (-20.7321, 1.95) -> (-17.2679, 1.95) projected
  line L4 (-17.2679, 1.95) -> (-15.5359, 4.95) projected
  line L5 (-15.5359, 4.95) -> (-17.2679, 7.95) projected
  line L6 (15.5359, 4.95) -> (17.2679, 1.95) projected
  line L7 (17.2679, 1.95) -> (20.7321, 1.95) projected
  line L8 (20.7321, 1.95) -> (22.4641, 4.95) projected
  line L9 (22.4641, 4.95) -> (20.7321, 7.95) projected
  line L10 (20.7321, 7.95) -> (17.2679, 7.95) projected
  line L11 (17.2679, 7.95) -> (15.5359, 4.95) projected
  circle A1 centre (19, 4.95) radius 1.75 projected
  point P0 (0, 0)
extrude "Wyciągnięcie proste24" cut sketch "Szkic25" against normal blind 2
sketch "Szkic26" plane through (0, 7, 0) normal (0, 1, 0) x (1, 0, 0)
  arc A0 (1.5, 18.2514) -> (-1.5, 18.2514) centre (0, 17.35) ccw projected
  line L0 (1.5, 18.2514) -> (1.5, 25) projected
  line L1 (1.5, 25) -> (-1.5, 25) projected
  line L2 (-1.5, 25) -> (-1.5, 18.2514) projected
  point P0 (0, 0)
extrude "Wyciągnięcie proste25" add sketch "Szkic26" along normal up to surface (1 mm away)
sketch "Szkic27" plane through (-25, 3, -9.7) normal (-1, 0, 0) x (0, 0, 1)
  line L0 (24.0847, 0) -> (23.5108, 4) projected
  line L1 (23.5108, 4) -> (23.5108, 5) projected
  line L2 (0, 5) -> (23.5108, 5) projected
  line L3 (0, 5) -> (0, 0) projected
  line L4 (0, 0) -> (24.0847, 0) projected
  line L5 (15.31, 5) -> (17.31, 5) projected
  line L6 (17.31, 5) -> (20.31, 5)
  line L7 (20.31, 5) -> (20.31, 9)
  line L8 (20.31, 9) -> (17.31, 9)
  line L9 (17.31, 9) -> (17.31, 5)
  line L10 (17.31, 5) -> (14.31, 5)
  line L11 (14.31, 5) -> (14.31, 9)
  line L12 (14.31, 9) -> (17.31, 9)
  line L13 (17.31, 9) -> (17.31, 5)
  circle A0 centre (17.31, 7) radius 1.5
  circle A1 centre (17.31, 7) radius 2
  line L14 (15.31, 7) -> (15.31, 5)
  line L15 (19.31, 7) -> (19.31, 5)
  point P0 (9.7, -3)
  dimension "d86" = 3
  dimension "d87" = 3
  dimension "d88" = 4
  dimension "d89" = 3
  constraints: 20 end point, 4 parallel, 3 perpendicular, 3 point on circle, 2 centre point, 2 horizontal, 2 point on line, 2 tangent, 1 coincident, 1 midpoint
  measures "d86" distance of L8.end L7.end
  measures "d87" distance of L11.end L12.end
  measures "d88" distance of L10.end L11.end
  measures "d89" diameter of A0
extrude "Wyciągnięcie proste26" add sketch "Szkic27" against normal blind 5 contours L2 A1 L15 | L14 A1 L2 | A1 L9 A0 | L9 A0 A1
fillet "Zaokrąglenie3" radius 1.5 2 edges at (-22.5, 8, 9.61) (-22.5, 8, 5.61)
sketch "Szkic28" plane through (-25, 3, -9.7) normal (-1, 0, 0) x (0, 0, 1)
  circle A0 centre (17.31, 7) radius 1.5 projected
  line L0 (24.0847, 0) -> (23.5108, 4) projected
  line L1 (23.5108, 4) -> (23.5108, 5) projected
  line L2 (20.81, 5) -> (23.5108, 5) projected
  arc A1 (19.31, 6.5) -> (20.81, 5) centre (20.81, 6.5) ccw projected
  line L3 (19.31, 6.5) -> (19.31, 7) projected
  arc A2 (19.31, 7) -> (15.31, 7) centre (17.31, 7) ccw projected
  line L4 (15.31, 7) -> (15.31, 6.5) projected
  arc A3 (13.81, 5) -> (15.31, 6.5) centre (13.81, 6.5) ccw projected
  line L5 (0, 5) -> (13.81, 5) projected
  line L6 (0, 5) -> (0, 0) projected
  line L7 (0, 0) -> (24.0847, 0) projected
  line L8 (13.81, 5) -> (20.81, 5)
  point P0 (9.7, -3)
  constraints: 2 end point, 1 collinear
extrude "Wyciągnięcie proste27" cut sketch "Szkic28" against normal blind 2 contours L8 A3 L4 A2 L3 A1
ref_plane "Płaszczyzna konstrukcyjna2" through (0, 3, -9.7) normal (-1, 0, 0) x (0, 0, 1)
mirror "Odbij1" about plane through (0, 3, -9.7) normal (-1, 0, 0) of "Wyciągnięcie proste27", "Zaokrąglenie3", "Wyciągnięcie proste26"
body "Solid1"
